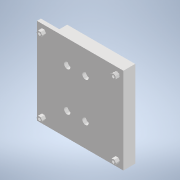
# Autodesk Inventor part: STM_Front
Saved by Autodesk Inventor 2020 (Build 240168000, 168)
## iProperties
Created: 2022-10-11
Part Number: STM_Front
Material: 일반
Document SubType Name: Modeling
Designer: ASUS
Mass: 207.503 g
Surface Area: 377.524 cm^2
Volume: 207.503 cm^3
Density: 1 g/cm^3
Appearance: 기본값
Author: ASUS
Autodesk Inventor part; units mm, degrees
ref_plane "YZ Plane" through (0, 0, 0) normal (1, 0, 0) x (0, 1, 0)
ref_plane "XZ Plane" through (0, 0, 0) normal (0, 1, 0) x (-1, 0, 0)
sketch "스케치1" plane through (0, 0, 0) normal (0, 0, 1) x (1, 0, 0)
  line L0 (-85, -210.5) -> (25, -210.5)
  line L1 (25, -210.5) -> (25, -100.5)
  line L2 (25, -100.5) -> (-85, -100.5)
  line L3 (-85, -100.5) -> (-85, -210.5)
  line L4 (-93.66, -289.5118) -> (-93.66, -125.5) projected
  line L5 (-28.54, -155.5) -> (-136.0279, -155.5) projected
  line L6 (25, 0) -> (25, -311) projected
  point P0 (0, 0)
  point P1 (-85, -155.5)
  dimension "d0" = 110
  dimension "d1" = 110
  constraints: 8 end point, 2 parallel, 1 collinear, 1 horizontal, 1 midpoint, 1 perpendicular, 1 point on line
  measures "d0" distance of L0.end L1.end
  measures "d1" distance of L1.end L2.end
extrude "돌출1" add sketch "스케치1" along normal blind 15
sketch "스케치2" plane through (0, 0, 0) normal (0, 0, -1) x (-1, 0, 0)
  line L0 (61.5, -115.5) -> (-388.5, -115.5) projected
  line L1 (61.5, -145.5) -> (-388.5, -145.5) projected
  line L2 (61.5, -165.5) -> (-388.5, -165.5) projected
  line L3 (61.5, -195.5) -> (-388.5, -195.5) projected
  line L4 (0, 0) -> (0, -311) projected
  line L5 (61.5, -195.5) -> (0, -195.5)
  line L6 (0, -195.5) -> (0, -165.5)
  line L7 (0, -165.5) -> (61.5, -165.5)
  line L8 (61.5, -165.5) -> (61.5, -195.5)
  line L9 (61.5, -145.5) -> (0, -145.5)
  line L10 (0, -145.5) -> (0, -115.5)
  line L11 (0, -115.5) -> (61.5, -115.5)
  line L12 (61.5, -115.5) -> (61.5, -145.5)
  point P0 (0, -195.5)
  point P1 (0, -145.5)
  constraints: 16 end point, 4 parallel, 4 point on line, 2 horizontal, 2 perpendicular
ref_plane "작업 평면1" through (-61.5, -145.5, -15) normal (0, 0, 1) x (1, 0, 0)
extrude "돌출2" add sketch "스케치2" along normal up to surface (15 mm away)
sketch "스케치3" plane through (-85, -210.5, 0) normal (-1, 0, 0) x (0, 0, 1)
  line L0 (-5, 71) -> (-5, 85) projected
  line L1 (-5, 85) -> (15, 85) projected
  line L2 (15, -79.0118) -> (15, 85) projected
  line L3 (-15, -79.0118) -> (15, -79.0118) projected
  line L4 (-15, 71) -> (-15, -79.0118) projected
  line L5 (-15, 71) -> (-5, 71) projected
  line L6 (5.5, 61.25) -> (-5.5, 61.25) projected
  line L7 (-5.5, 61.25) -> (-5.5, 58.75) projected
  line L8 (-5.5, 58.75) -> (5.5, 58.75) projected
  line L9 (5.5, 58.75) -> (5.5, 61.25) projected
  line L10 (-5.5, 48.75) -> (5.5, 48.75) projected
  line L11 (5.5, 48.75) -> (5.5, 51.25) projected
  line L12 (5.5, 51.25) -> (-5.5, 51.25) projected
  line L13 (-5.5, 51.25) -> (-5.5, 48.75) projected
  line L14 (0, 110) -> (15, 110) projected
  line L15 (0, 0) -> (15, 0) projected
  line L16 (15, 110) -> (10, 110)
  line L17 (10, 110) -> (10, 0)
  line L18 (10, 0) -> (15, 0)
  line L19 (15, 0) -> (15, 110)
  line L20 (0, 110) -> (0, 0) projected
  point P0 (0, 210.5)
  point P1 (10, 110)
  dimension "d7" = 5
  constraints: 8 end point, 2 parallel, 1 horizontal, 1 perpendicular, 1 point on line
  measures "d7" distance between parallel lines of L2 L17
extrude "돌출3" cut sketch "스케치3" against normal up to surface (23.5 mm away) contours L20 L14 L17 L1 | L1 L17 L15 L20 L10 L11 L12 L8 L9 L6 | L6 L9 L8 L20 | L12 L11 L10 L20
sketch "스케치4" plane through (0, 0, 15) normal (0, 0, 1) x (1, 0, 0)
  circle A0 centre (-46.5, -180.5) radius 4 projected
  circle A1 centre (-46.5, -130.5) radius 4 projected
  line L0 (0, 0) -> (0, -311) projected
  line L1 (-46.5, -180.5) -> (0, -180.5)
  line L2 (-46.5, -130.5) -> (0, -130.5)
  line L3 (0, -145.5) -> (0, -115.5) projected
  point P0 (-23.25, -130.5)
  point P1 (-23.25, -180.5)
  constraints: 4 end point, 3 midpoint, 1 perpendicular, 1 point on line
hole "구멍1" at (-23.25, -180.5, 15) at (-23.25, -130.5, 15) at (-46.5, -130.5, 15) at (-46.5, -180.5, 15) direction (0, 0, -1) diameter 4.5 end through all counterbore diameter 8 counterbore depth 4.6 clearance for "Socket Head Cap Screw ISO 4762" size "M4" standard "ISO"
sketch "스케치7" plane through (-85, -210.5, 10) normal (0, 0, -1) x (-1, 0, 0)
  line L0 (0, 0) -> (-23.5, 0) projected
  line L1 (0, 110) -> (0, 0) projected
  line L2 (-23.5, 110) -> (0, 110) projected
  circle A0 centre (-8, 8) radius 3
  circle A1 centre (-8, 102) radius 3
  line L3 (-9.7321, 99) -> (-11.4641, 102)
  line L4 (-11.4641, 102) -> (-9.7321, 105)
  line L5 (-9.7321, 105) -> (-6.2679, 105)
  line L6 (-6.2679, 105) -> (-4.5359, 102)
  line L7 (-4.5359, 102) -> (-6.2679, 99)
  line L8 (-6.2679, 99) -> (-9.7321, 99)
  line L9 (-9.7321, 5) -> (-11.4641, 8)
  line L10 (-11.4641, 8) -> (-9.7321, 11)
  line L11 (-9.7321, 11) -> (-6.2679, 11)
  line L12 (-6.2679, 11) -> (-4.5359, 8)
  line L13 (-4.5359, 8) -> (-6.2679, 5)
  line L14 (-6.2679, 5) -> (-9.7321, 5)
  point P0 (-85, 210.5)
  point P1 (-8, 99)
  point P2 (-8, 5)
  dimension "d28" = 6
  dimension "d29" = 6
  dimension "d25" = 8
  dimension "d26" = 8
  dimension "d27" = 8
  constraints: 24 end point, 4 coincident, 3 vertical alignment, 2 midpoint, 30 other
  measures "d25" distance from line of L0 point (-8, 8)
  measures "d26" distance from line of L1 point (-8, 8)
  measures "d27" distance from line of L2 point (-8, 102)
extrude "돌출4" cut sketch "스케치7" against normal blind 3
sketch "스케치9" plane through (0, 0, 0) normal (0, 0, -1) x (-1, 0, 0)
  line L0 (61.5, -210.5) -> (61.5, -195.5) projected
  line L1 (61.5, -195.5) -> (0, -195.5) projected
  line L2 (0, -195.5) -> (0, -165.5) projected
  line L3 (0, -165.5) -> (61.5, -165.5) projected
  line L4 (61.5, -165.5) -> (61.5, -145.5) projected
  line L5 (61.5, -145.5) -> (0, -145.5) projected
  line L6 (0, -145.5) -> (0, -115.5) projected
  line L7 (0, -115.5) -> (61.5, -115.5) projected
  line L8 (61.5, -115.5) -> (61.5, -100.5) projected
  line L9 (-25, -100.5) -> (61.5, -100.5) projected
  line L10 (-25, -210.5) -> (-25, -100.5) projected
  line L11 (61.5, -210.5) -> (-25, -210.5) projected
  circle A0 centre (-17, -202.5) radius 3
  circle A1 centre (-17, -108.5) radius 3
  line L12 (-13.8603, -107.0363) -> (-14.1626, -110.4872)
  line L13 (-14.1626, -110.4872) -> (-17.3022, -111.9509)
  line L14 (-17.3022, -111.9509) -> (-20.1397, -109.9637)
  line L15 (-20.1397, -109.9637) -> (-19.8374, -106.5128)
  line L16 (-19.8374, -106.5128) -> (-16.6978, -105.0491)
  line L17 (-16.6978, -105.0491) -> (-13.8603, -107.0363)
  line L18 (-14.9745, -199.6898) -> (-13.5535, -202.849)
  line L19 (-13.5535, -202.849) -> (-15.579, -205.6592)
  line L20 (-15.579, -205.6592) -> (-19.0255, -205.3102)
  line L21 (-19.0255, -205.3102) -> (-20.4465, -202.151)
  line L22 (-20.4465, -202.151) -> (-18.421, -199.3408)
  line L23 (-18.421, -199.3408) -> (-14.9745, -199.6898)
  point P0 (0, 0)
  point P1 (-15.279, -106.0427)
  point P2 (-16.6978, -199.5153)
  dimension "d32" = 6
  dimension "d36" = 6
  dimension "d33" = 8
  dimension "d34" = 8
  dimension "d35" = 8
  constraints: 24 end point, 2 coincident, 2 midpoint, 1 vertical alignment, 32 other
  measures "d33" distance from line of L9 point (-17, -108.5)
  measures "d34" distance from line of L10 point (-17, -108.5)
  measures "d35" distance from line of L11 point (-17, -202.5)
extrude "돌출5" cut sketch "스케치9" against normal blind 5 contours A0 | A0 L18 L19 | A0 L23 L18 | L19 L20 A0 | A0 L22 L23 | L20 L21 A0 | A0 L21 L22 | A1 | A1 L17 L12 | A1 L16 L17 | L12 L13 A1 | A1 L15 L16 | L13 L14 A1 | A1 L14 L15
sketch "스케치10" plane through (0, 0, 15) normal (0, 0, 1) x (1, 0, 0)
  line L0 (-75.2679, -105.5) -> (-78.7321, -105.5) projected
  line L1 (-78.7321, -105.5) -> (-80.4641, -108.5) projected
  line L2 (-80.4641, -108.5) -> (-78.7321, -111.5) projected
  line L3 (-78.7321, -111.5) -> (-75.2679, -111.5) projected
  line L4 (-75.2679, -111.5) -> (-73.5359, -108.5) projected
  line L5 (-73.5359, -108.5) -> (-75.2679, -105.5) projected
  line L6 (-78.7321, -199.5) -> (-80.4641, -202.5) projected
  line L7 (-80.4641, -202.5) -> (-78.7321, -205.5) projected
  line L8 (-78.7321, -205.5) -> (-75.2679, -205.5) projected
  line L9 (-75.2679, -205.5) -> (-73.5359, -202.5) projected
  line L10 (-73.5359, -202.5) -> (-75.2679, -199.5) projected
  line L11 (-75.2679, -199.5) -> (-78.7321, -199.5) projected
  line L12 (-61.5, -100.5) -> (-61.5, -210.5) projected
  line L13 (-85, -210.5) -> (-61.5, -210.5) projected
  line L14 (-85, -100.5) -> (-85, -210.5) projected
  line L15 (-61.5, -100.5) -> (-85, -100.5) projected
  line L16 (14.1626, -110.4872) -> (17.3022, -111.9509) projected
  line L17 (17.3022, -111.9509) -> (20.1397, -109.9637) projected
  line L18 (20.1397, -109.9637) -> (19.8374, -106.5128) projected
  line L19 (19.8374, -106.5128) -> (16.6978, -105.0491) projected
  line L20 (16.6978, -105.0491) -> (13.8603, -107.0363) projected
  line L21 (13.8603, -107.0363) -> (14.1626, -110.4872) projected
  line L22 (13.5535, -202.849) -> (15.579, -205.6592) projected
  line L23 (15.579, -205.6592) -> (19.0255, -205.3102) projected
  line L24 (19.0255, -205.3102) -> (20.4465, -202.151) projected
  line L25 (20.4465, -202.151) -> (18.421, -199.3408) projected
  line L26 (18.421, -199.3408) -> (14.9745, -199.6898) projected
  line L27 (14.9745, -199.6898) -> (13.5535, -202.849) projected
  line L28 (-61.5, -210.5) -> (-61.5, -195.5) projected
  line L29 (-61.5, -195.5) -> (0, -195.5) projected
  line L30 (0, -195.5) -> (0, -165.5) projected
  line L31 (0, -165.5) -> (-61.5, -165.5) projected
  line L32 (-61.5, -165.5) -> (-61.5, -145.5) projected
  line L33 (-61.5, -145.5) -> (0, -145.5) projected
  line L34 (0, -145.5) -> (0, -115.5) projected
  line L35 (0, -115.5) -> (-61.5, -115.5) projected
  line L36 (-61.5, -115.5) -> (-61.5, -100.5) projected
  line L37 (25, -100.5) -> (-61.5, -100.5) projected
  line L38 (25, -210.5) -> (25, -100.5) projected
  line L39 (-61.5, -210.5) -> (25, -210.5) projected
  point P0 (0, 0)
extrude "돌출6" add sketch "스케치10" along normal blind 5 contours L5 L4 L3 L2 L1 L0 | L11 L10 L9 L8 L7 L6 | L21 L20 L19 L18 L17 L16 | L27 L26 L25 L24 L23 L22
sketch "스케치11" plane through (0, 0, 20) normal (0, 0, 1) x (1, 0, 0)
  line L0 (20.1397, -109.9637) -> (17.3022, -111.9509) projected
  line L1 (17.3022, -111.9509) -> (14.1626, -110.4872) projected
  line L2 (14.1626, -110.4872) -> (13.8603, -107.0363) projected
  line L3 (13.8603, -107.0363) -> (16.6978, -105.0491) projected
  line L4 (16.6978, -105.0491) -> (19.8374, -106.5128) projected
  line L5 (19.8374, -106.5128) -> (20.1397, -109.9637) projected
  line L6 (20.4465, -202.151) -> (19.0255, -205.3102) projected
  line L7 (19.0255, -205.3102) -> (15.579, -205.6592) projected
  line L8 (15.579, -205.6592) -> (13.5535, -202.849) projected
  line L9 (13.5535, -202.849) -> (14.9745, -199.6898) projected
  line L10 (14.9745, -199.6898) -> (18.421, -199.3408) projected
  line L11 (18.421, -199.3408) -> (20.4465, -202.151) projected
  line L12 (-75.2679, -105.5) -> (-73.5359, -108.5) projected
  line L13 (-73.5359, -108.5) -> (-75.2679, -111.5) projected
  line L14 (-75.2679, -111.5) -> (-78.7321, -111.5) projected
  line L15 (-78.7321, -111.5) -> (-80.4641, -108.5) projected
  line L16 (-80.4641, -108.5) -> (-78.7321, -105.5) projected
  line L17 (-78.7321, -105.5) -> (-75.2679, -105.5) projected
  line L18 (-75.2679, -205.5) -> (-78.7321, -205.5) projected
  line L19 (-78.7321, -205.5) -> (-80.4641, -202.5) projected
  line L20 (-80.4641, -202.5) -> (-78.7321, -199.5) projected
  line L21 (-78.7321, -199.5) -> (-75.2679, -199.5) projected
  line L22 (-75.2679, -199.5) -> (-73.5359, -202.5) projected
  line L23 (-73.5359, -202.5) -> (-75.2679, -205.5) projected
  circle A0 centre (-46.5, -130.5) radius 4 projected
  circle A1 centre (-23.25, -180.5) radius 4 projected
  circle A2 centre (-23.25, -130.5) radius 4 projected
  circle A3 centre (-46.5, -180.5) radius 4 projected
  line L24 (-85, -210.5) -> (25, -210.5) projected
  line L25 (25, -210.5) -> (25, -100.5) projected
  line L26 (25, -100.5) -> (-85, -100.5) projected
  line L27 (-85, -100.5) -> (-85, -210.5) projected
  circle A4 centre (17, -202.5) radius 3
  circle A5 centre (-77, -202.5) radius 3
  circle A6 centre (-77, -108.5) radius 3
  circle A7 centre (17, -108.5) radius 3
  point P0 (0, 0)
  constraints: 12 tangent, 4 centre point
hole "구멍2" at (17, -108.5, 20) at (-77, -108.5, 20) at (-77, -202.5, 20) at (17, -202.5, 20) direction (0, 0, -1) diameter 3.4 end through all clearance for "Hex Head Cap Screw ISO 24017" size "M3" standard "ISO"
